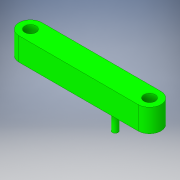
# Autodesk Inventor part: arm
Saved by Autodesk Inventor 2016 (Build 200138000, 138)
## iProperties
Created: 2018-01-12
Part Number: arm
Material: Aluminum 6061
Document SubType Name: Modeling
Designer: New User
Density: 2.7 g/cm^3
Appearance: Aluminum - Flat
Mass: 1109.3 g
Surface Area: 532.958 cm^2
Volume: 410.85 cm^3
Author: New User
Autodesk Inventor part; units mm, degrees
ref_plane "YZ Plane" through (0, 0, 0) normal (1, 0, 0) x (0, 1, 0)
ref_plane "XZ Plane" through (0, 0, 0) normal (0, 1, 0) x (-1, 0, 0)
ref_plane "XY Plane" through (0, 0, 0) normal (0, 0, 1) x (1, 0, 0)
sketch "Sketch1" plane through (0, 0, 0) normal (0, 1, 0) x (-1, 0, 0)
  line L0 (0, 0) -> (-25.4, 0)
  line L1 (-25.4, -152.4) -> (-157.48, -152.4)
  line L2 (-157.48, -152.4) -> (-157.48, -177.8)
  line L3 (-157.48, -177.8) -> (0, -177.8)
  line L4 (0, -177.8) -> (0, -152.4)
  line L5 (-25.4, -152.4) -> (0, -152.4)
  dimension "d2" = 25.4
  dimension "d23" = 157.48
  constraints: 12 end point, 5 perpendicular, 1 horizontal
  measures "d2" distance of L1.end L2.end
  measures "d23" distance of L2.end L3.end
extrude "Extrusion1" add sketch "Sketch1" along normal blind 25.4
sketch "Sketch2" plane through (0, 25.4, 0) normal (0, 1, 0) x (1, 0, 0)
  circle A0 centre (144.78, 165.1) radius 6.35
  line L0 (157.48, 152.4) -> (157.48, 177.8) projected
  line L1 (157.48, 177.8) -> (0, 177.8) projected
  circle A1 centre (12.7, 165.1) radius 6.35
  line L2 (0, 152.4) -> (157.48, 152.4) projected
  line L3 (0, 177.8) -> (0, 152.4) projected
  point P0 (0, 0)
  dimension "d5" = 12.7
  dimension "d6" = 12.7
  dimension "d7" = 12.7
  dimension "d16" = 12.7
  dimension "d17" = 12.7
  constraints: 2 centre point, 1 equal radius
  measures "d5" diameter of A0
  measures "d6" distance from line of L0 A0.centre
  measures "d7" distance from line of L1 A0.centre
  measures "d16" distance from line of L2 A1.centre
  measures "d17" distance from line of L3 A1.centre
extrude "Extrusion2" cut sketch "Sketch2" against normal blind 41.275 contours A0 | A1
fillet "Fillet1" radius 12.7 4 edges at (157.48, 12.7, -152.4) (157.48, 12.7, -177.8) (0, 12.7, -152.4) (0, 12.7, -177.8)
sketch "Sketch4" plane through (0, 0, 0) normal (0, -1, 0) x (1, 0, 0)
  circle A0 centre (106.68, -165.1) radius 3.175
  line L0 (144.78, -177.8) -> (12.7, -177.8) projected
  circle A1 centre (144.78, -165.1) radius 6.35 projected
  point P0 (0, 0)
  dimension "d18" = 6.35
  dimension "d19" = 12.7
  dimension "d20" = 38.1
  constraints: 1 centre point
  measures "d18" diameter of A0
  measures "d19" distance from line of L0 A0.centre
  measures "d20" distance of A1.centre A0.centre
extrude "Extrusion4" add sketch "Sketch4" along normal blind 25.4 contours A0
body "Solid1"
